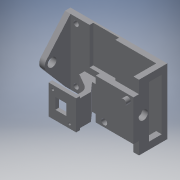
# Autodesk Inventor part: LPATFORM
Saved by Autodesk Inventor 2019 (Build 230136000, 136)
## iProperties
Created: 2020-03-28
Part Number: LPATFORM
Material: Generic
Document SubType Name: Modeling
Designer: Pulag
Density: 1 g/cm^3
Appearance: Default
Author: Pulag
Autodesk Inventor part; units mm, degrees
ref_plane "YZ Plane" through (0, 0, 0) normal (1, 0, 0) x (0, 1, 0)
ref_plane "XZ Plane" through (0, 0, 0) normal (0, 1, 0) x (-1, 0, 0)
ref_plane "XY Plane" through (0, 0, 0) normal (0, 0, 1) x (1, 0, 0)
sketch "Sketch1" plane through (0, 0, 0) normal (1, 0, 0) x (0, 1, 0)
  circle A0 centre (1.0813, 17.8439) radius 2.5
  line L0 (18.8613, 4.8439) -> (18.8613, 7.8439)
  line L1 (18.8613, 7.8439) -> (-16.6987, 7.8439)
  line L2 (-16.6987, 4.8439) -> (-16.6987, 7.8439)
  circle A1 centre (1.0813, 17.8439) radius 4
  line L3 (-16.6987, 4.8439) -> (18.8613, 4.8439)
  line L4 (-9.9187, 25.1972) -> (12.0813, 25.1972) projected
  line L5 (12.0813, 25.1972) -> (12.0813, 23.1972) projected
  line L6 (-9.9187, 23.1972) -> (12.0813, 23.1972) projected
  line L7 (-9.9187, 25.1972) -> (-9.9187, 23.1972) projected
  line L8 (-9.9187, 23.1972) -> (12.0813, 23.1972)
  line L9 (1.0813, 7.8439) -> (15.0813, 7.8439)
  line L10 (15.0813, 7.8439) -> (15.0813, 14.8439)
  line L11 (15.0813, 14.8439) -> (1.0813, 14.8439)
  line L12 (1.0813, 7.8439) -> (-12.9187, 7.8439)
  line L13 (-12.9187, 7.8439) -> (-12.9187, 14.8439)
  line L14 (-12.9187, 14.8439) -> (1.0813, 14.8439)
  line L15 (12.0813, 23.1972) -> (18.8613, 23.1972)
  line L16 (18.8613, 23.1972) -> (18.8613, 7.8439)
  line L17 (-9.9187, 23.1972) -> (-16.6987, 23.1972)
  line L18 (-16.6987, 23.1972) -> (-16.6987, 7.8439)
  line L19 (-12.9187, 14.8439) -> (15.0813, 14.8439)
  line L20 (15.0813, 14.8439) -> (15.0813, 7.8439)
  line L21 (15.0813, 7.8439) -> (-12.9187, 7.8439)
  line L22 (-12.9187, 7.8439) -> (-12.9187, 14.8439)
  dimension "d0" = 5
  dimension "d21" = 35.56
  dimension "d25" = 3
  dimension "d27" = 8
  dimension "d41" = 14
  dimension "d42" = 7
  dimension "d43" = 14
  constraints: 38 end point, 7 perpendicular, 5 equal length, 4 horizontal, 2 centre point, 2 point on line, 1 concentric, 1 midpoint, 1 vertical
  measures "d0" diameter of A0
  measures "d21" distance of L2.start L0.start
  measures "d25" distance of L0.start L0.end
  measures "d27" diameter of A1
  measures "d41" distance of L11.end L10.end
  measures "d42" distance of L10.end L9.end
  measures "d43" distance of L13.end L14.end
extrude "Extrusion1" add sketch "Sketch1" against normal blind 3 contours L3 L2 L1 L0 | L1 L10 L11 A1 L14 L13 L18 L17 L6 L15 L16 | L11 L14 A1 picked at (-0.0961, 15.0647)
sketch "Sketch3" plane through (-3, 0, 0) normal (-1, 0, 0) x (0, 0, 1)
  line L0 (4.8439, -16.6987) -> (4.8439, 7.1463)
  line L1 (4.8439, 18.2263) -> (4.8439, 7.1463)
  line L2 (4.8439, -16.6987) -> (7.8439, -16.6987)
  line L3 (7.8439, -16.6987) -> (7.8439, 18.8613)
  line L4 (7.8439, 18.8613) -> (4.8439, 18.8613)
  line L5 (4.8439, 18.8613) -> (4.8439, -16.6987)
  circle A0 centre (17.8439, 1.0813) radius 2.5 projected
  line L6 (4.8439, -16.6987) -> (23.1972, -16.6987) projected
  line L7 (23.1972, 18.8613) -> (4.8439, 18.8613) projected
  line L8 (4.8439, 18.8613) -> (4.8439, -16.6987) projected
  line L9 (23.1972, -16.6987) -> (23.1972, 18.8613) projected
  point P0 (0, 0)
  point P1 (7.8439, 1.0813)
  dimension "d8" = 3
  dimension "d9" = 35.56
  constraints: 12 end point, 2 parallel, 1 horizontal, 1 midpoint, 1 perpendicular
  measures "d8" distance of L4.end L3.end
  measures "d9" distance of L2.end L3.end
ref_plane "Work Plane1" through (-49.2583, -17.4787, 7.8439) normal (-1, 0, 0) x (0, 0, 1)
ref_plane "Work Plane2" through (-49.5083, -6.4187, 16.0439) normal (-1, 0, 0) x (0, 0, 1)
extrude "Extrusion2" add sketch "Sketch3" along normal up to surface (46.5083 mm away) contours L0 L1 L5 L4 L3 L2
sketch "Sketch4" plane through (-3, 18.8613, 7.8439) normal (0, 1, 0) x (1, 0, 0)
  line L0 (0, 0) -> (-46.5083, 0) projected
  line L1 (-36.1522, 0) -> (-22.1522, 0)
  line L2 (-22.1522, 0) -> (-22.1522, 2)
  line L3 (-22.1522, 2) -> (-36.1522, 2)
  line L4 (-36.1522, 2) -> (-36.1522, 0)
  line L5 (-29.1522, 0) -> (-29.1522, 2)
  point P0 (3, 7.8439)
  point P1 (-52, 0)
  dimension "d14" = 2
  dimension "d19" = 7
  dimension "d20" = 7
  constraints: 10 end point, 2 midpoint, 2 parallel, 1 horizontal, 1 perpendicular, 1 point on line, 1 vertical
  measures "d14" distance of L1.end L2.end
  measures "d19" distance between parallel lines of L5 L2
  measures "d20" distance between parallel lines of L4 L5
extrude "Extrusion3" cut sketch "Sketch4" against normal blind 20
sketch "Sketch7" plane through (-49.5083, -16.6987, 4.8439) normal (-1, 0, 0) x (0, 0, 1)
  line L0 (3, 0) -> (16.0342, 15.1736) projected
  arc A0 (16.0342, 15.1736) -> (16.0342, 20.3864) centre (13, 17.78) ccw projected
  line L1 (16.0342, 20.3864) -> (3, 35.56) projected
  circle A1 centre (13, 17.78) radius 2.4 projected
  line L2 (0, 0) -> (0, 35.56) projected
  line L3 (3, 0) -> (0, 0) projected
  line L4 (0, 35.56) -> (3, 35.56) projected
  point P0 (-4.8439, 16.6987)
extrude "Extrusion5" add sketch "Sketch7" along normal blind 3
sketch "Sketch8" plane through (-3, -16.6987, 7.8439) normal (0, 0, 1) x (1, 0, 0)
  line L0 (-7.4083, 8.61) -> (-9.4083, 8.61)
  line L1 (-9.4083, 8.61) -> (-9.4083, 5.61)
  line L2 (-9.4083, 5.61) -> (-7.4083, 5.61)
  line L3 (-7.4083, 5.61) -> (-7.4083, 8.61)
  line L4 (-7.4083, 8.61) -> (-9.4083, 5.61) construction
  line L5 (-9.4083, 8.61) -> (-7.4083, 5.61) construction
  point P0 (3, 16.6987)
  point P1 (-8.4083, 7.11)
  dimension "d82" = 2
  dimension "d83" = 3
  constraints: 12 end point, 2 midpoint, 2 parallel, 1 horizontal, 1 perpendicular
  measures "d82" distance of L2.end L1.end
  measures "d83" distance of L1.end L0.end
extrude "Extrusion6" cut sketch "Sketch8" against normal blind 3
sketch "Sketch9" plane through (-3, 0, 0) normal (-1, 0, 0) x (0, 0, 1)
  line L0 (7.8439, -16.6987) -> (23.1972, -16.6987) projected
  line L1 (23.1972, 18.911) -> (20.1972, 18.911)
  line L2 (20.1972, 18.911) -> (20.1972, -16.6987)
  line L3 (20.1972, -16.6987) -> (23.1972, -16.6987)
  line L4 (23.1972, -16.6987) -> (23.1972, 18.911)
  point P0 (0, 0)
  dimension "d45" = 3
  constraints: 8 end point, 2 parallel, 1 horizontal, 1 perpendicular, 1 point on line
  measures "d45" distance of L3.end L2.end
extrude "Extrusion7" add sketch "Sketch9" along normal blind 26.5
sketch "Sketch10" plane through (0, -16.6987, 23.1972) normal (0, 0, 1) x (1, 0, 0)
  line L0 (-20.4523, 28.78) -> (-0.4523, 28.78) projected
  line L1 (-20.4523, 6.78) -> (-20.4523, 28.78) projected
  line L2 (-0.4523, 6.78) -> (-20.4523, 6.78) projected
  line L3 (-20.5843, 10.78) -> (-32.0843, 10.78) projected
  line L4 (-32.0843, 24.78) -> (-20.5843, 24.78) projected
  line L5 (-20.4523, 24.78) -> (-29.5, 24.78)
  line L6 (-29.5, 24.78) -> (-29.5, 35.6097)
  line L7 (-29.5, 35.6097) -> (-20.4523, 35.6097)
  line L8 (-20.4523, 35.6097) -> (-20.4523, 24.78)
  line L9 (-20.4523, 28.78) -> (0, 28.78)
  line L10 (0, 28.78) -> (0, 35.6097)
  line L11 (0, 35.6097) -> (-20.4523, 35.6097)
  line L12 (-20.4523, 35.6097) -> (-20.4523, 28.78)
  line L13 (-29.5, 0) -> (-20.4523, 0)
  line L14 (-20.4523, 0) -> (-20.4523, 10.78)
  line L15 (-20.4523, 10.78) -> (-29.5, 10.78)
  line L16 (-29.5, 10.78) -> (-29.5, 0)
  line L17 (-20.4523, 6.78) -> (0, 6.78)
  line L18 (0, 6.78) -> (0, 0)
  line L19 (0, 0) -> (-20.4523, 0)
  line L20 (-20.4523, 0) -> (-20.4523, 6.78)
  constraints: 32 end point, 8 parallel, 5 point on line, 4 horizontal, 4 perpendicular
extrude "Extrusion8" cut sketch "Sketch10" against normal blind 3
sketch "Sketch11" plane through (0, -9.9187, 23.1972) normal (0, 0, 1) x (1, 0, 0)
  line L0 (-19.5843, 3) -> (-33.0843, 3)
  line L1 (-33.0843, 3) -> (-33.0843, 19)
  line L2 (-33.0843, 19) -> (-19.5843, 19)
  line L3 (-19.5843, 19) -> (-19.5843, 3)
  line L4 (-19.5843, 3) -> (-33.0843, 19) construction
  line L5 (-33.0843, 3) -> (-19.5843, 19) construction
  line L6 (-23.0843, 7.75) -> (-29.5843, 7.75)
  line L7 (-29.5843, 7.75) -> (-29.5843, 14.25)
  line L8 (-29.5843, 14.25) -> (-23.0843, 14.25)
  line L9 (-23.0843, 14.25) -> (-23.0843, 7.75)
  line L10 (-23.0843, 7.75) -> (-29.5843, 14.25) construction
  line L11 (-29.5843, 7.75) -> (-23.0843, 14.25) construction
  circle A0 centre (-30.8843, 16.8) radius 1
  circle A1 centre (-21.7843, 5.2) radius 1
  point P0 (0, 9.9187)
  point P1 (-26.3343, 11)
  dimension "d50" = 13.5
  dimension "d51" = 16
  dimension "d76" = 6.5
  dimension "d77" = 6.5
  dimension "d78" = 2
  dimension "d79" = 2
  constraints: 24 end point, 4 midpoint, 4 parallel, 2 centre point, 2 horizontal, 2 perpendicular
  measures "d50" distance of L1.end L2.end
  measures "d51" distance of L0.end L1.end
  measures "d76" distance of L7.end L8.end
  measures "d77" distance of L6.end L7.end
  measures "d78" diameter of A0
  measures "d79" diameter of A1
ref_plane "Work Plane3" through (-32.0843, -5.9187, 34.1972) normal (0, 0, 1) x (1, 0, 0)
extrude "Extrusion9" add sketch "Sketch11" along normal blind 2 from surface at 11
sketch "Sketch12" plane through (-33.0843, 9.0813, 36.1972) normal (0, 1, 0) x (1, 0, 0)
  line L0 (12.5, 2) -> (13.5, 2)
  line L1 (13.5, 2) -> (13.5, 8)
  line L2 (12.7351, 7.8643) -> (12.7351, 2)
  line L3 (13.5, 8) -> (19.2735, 8) construction
  line L4 (12.5, 8) -> (3.8397, 13)
  line L5 (3.8397, 13) -> (10.6132, 13)
  line L6 (13.5, 8) -> (15, 8)
  line L7 (15, 8) -> (12, 11.4194)
  line L8 (12.5, 8) -> (12.7351, 7.8643)
  line L9 (13.5, 2) -> (12.7351, 2)
  line L10 (0, 2) -> (13.5, 2) projected
  line L11 (12.632, 11) -> (12.632, 13) projected
  line L12 (12, 13) -> (12, 11.4194)
  line L13 (12, 13) -> (3.8397, 13)
  line L14 (12.632, 13) -> (3.5843, 13) projected
  point P0 (33.0843, 36.1972)
  dimension "d54" = 6
  dimension "d58" = 120
  dimension "d67" = 1.5
  constraints: 24 end point, 3 horizontal, 2 collinear, 1 parallel, 1 perpendicular, 1 point on line, 1 vertical
  measures "d54" distance of L1.end L0.end
  measures "d58" angle of L4 L2
  measures "d67" distance of L1.end L6.end
extrude "Extrusion10" add sketch "Sketch12" along normal up to surface (14 mm away) from surface at -15
fillet "Fillet2" radius 5 1 edges at (-20.3492, 1.0813, 28.3329)
fillet "Fillet3" radius 3 1 edges at (-29.2446, 1.0813, 23.1972)
sketch "Sketch13" plane through (-3, -12.9187, 7.8439) normal (0, 0, 1) x (1, 0, 0)
  circle A0 centre (-43.4583, 28.73) radius 2
  circle A1 centre (-43.4583, -0.73) radius 2
  point P0 (3, 12.9187)
  dimension "d80" = 4
  dimension "d81" = 4
  constraints: 2 centre point
  measures "d80" diameter of A0
  measures "d81" diameter of A1
extrude "Extrusion11" cut sketch "Sketch13" against normal blind 3
sketch "Sketch15" plane through (0, -9.9187, 23.1972) normal (0, 0, 1) x (1, 0, 0)
  circle A0 centre (-3.0523, 19.4) radius 1.6 projected
  circle A1 centre (-15.8523, 2.6) radius 1.6 projected
  point P0 (0, 9.9187)
extrude "Extrusion13" cut sketch "Sketch15" against normal up to surface (3 mm away) contours A1
sketch "Sketch16" plane through (0, -9.9187, 23.1972) normal (0, 0, 1) x (1, 0, 0)
  circle A0 centre (-3.0523, 19.4) radius 1.6 projected
  point P0 (0, 9.9187)
ref_plane "Work Plane4" through (-20.4523, -9.9187, 25.1972) normal (0, 0, 1) x (1, 0, 0)
extrude "Extrusion14" add sketch "Sketch16" along normal blind 2.5
sketch "Sketch17" plane through (-19.5843, -6.9187, 36.1972) normal (1, 0, 0) x (0, 0, -1)
  line L0 (0, 16) -> (0, 0) projected
  line L1 (2, 0) -> (0, 0) projected
  line L2 (2, 1) -> (2, 0) projected
  line L3 (0, 16) -> (2, 16) projected
  line L4 (8, 1) -> (2, 1) projected
  line L5 (8, 15) -> (8, 1) projected
  line L6 (2, 15) -> (8, 15) projected
  line L7 (2, 16) -> (2, 15) projected
  point P0 (36.1972, 6.9187)
extrude "Extrusion15" add sketch "Sketch17" along normal blind 1.5
body "Solid1"
